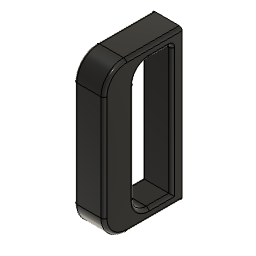
handle (Autodesk Fusion 360 design; units mm, degrees)
Autodesk Fusion 360 part; units mm, degrees
sketch "Sketch1" plane through (0, 0, 0) normal (1, 0, 0) x (0, 1, 0)
  line L0 (-66.04, 63.5) -> (0, 63.5)
  line L1 (0, 63.5) -> (0, -63.5)
  line L2 (0, -63.5) -> (-66.04, -63.5)
  line L3 (-66.04, -63.5) -> (-66.04, 63.5)
  line L4 (-8.89, 54.61) -> (-40.64, 54.61)
  line L5 (-40.64, 54.61) -> (-40.64, -54.61)
  line L6 (-40.64, -54.61) -> (-8.89, -54.61)
  line L7 (-8.89, -54.61) -> (-8.89, 54.61)
  dimension "d1" = 127
  dimension "d2" = 31.75
  dimension "d3" = 8.89
  dimension "d4" = 8.89
  dimension "d5" = 25.4
  dimension "d6" = 8.89
  constraint horizontal L0
  constraint vertical L1
  constraint horizontal L2
  constraint vertical L3
  constraint midpoint L1 origin
  constraint horizontal L4
  constraint vertical L5
  constraint horizontal L6
  constraint vertical L7
  measures "d1" distance of L0.end L1.end
  measures "d2" distance of L5 L7
  measures "d3" distance of L0 L4
  measures "d4" distance of L1 L7
  measures "d5" distance of L3 L5
  measures "d6" distance of L2 L6
extrude "Extrude1" add sketch "Sketch1" along normal mid plane 25.4
fillet "Fillet1" radius 12.7 1 edges at (0, -40.64, -54.61)
fillet "Fillet2" radius 12.7 1 edges at (0, -40.64, 54.61)
fillet "Fillet3" radius 19.05 1 edges at (0, -66.04, 63.5)
fillet "Fillet4" radius 19.05 1 edges at (0, -66.04, -63.5)
sketch "Sketch2" plane through (0, -66.04, 0) normal (0, -1, 0) x (1, 0, 0)
  line L0 (-12.7, -44.45) -> (12.7, -44.45)
  line L1 (12.7, -44.45) -> (12.7, 44.45)
  line L2 (12.7, 44.45) -> (-12.7, 44.45)
  line L3 (-12.7, 44.45) -> (-12.7, -44.45)
  line L4 (7.181, -50.5634) -> (7.181, 50.5634) construction
  line L5 (7.181, 50.5634) -> (-7.181, 50.5634) construction
  line L6 (-7.181, 50.5634) -> (-7.181, -50.5634) construction
  line L7 (-7.181, -50.5634) -> (7.181, -50.5634) construction
  dimension "d17" = 12.7
  constraint vertical L6
  constraint horizontal origin
  constraint vertical origin
extrude "Extrude2" [suppressed]
fillet "Fillet5" radius 2.5 23 edges at (12.7, -8.89, 0) (0, -8.89, 54.61) (12.7, -18.415, -54.61) (12.7, -36.9203, -50.8903) (12.7, -40.64, 0) (12.7, -36.9203, 50.8903) (12.7, -18.415, 54.61) (-12.7, -8.89, 0) (-12.7, -18.415, 54.61) (-12.7, -36.9203, 50.8903) (-12.7, -40.64, 0) (-12.7, -36.9203, -50.8903) (-12.7, -18.415, -54.61) (12.7, -23.495, 63.5) (12.7, -60.4604, 57.9204) (12.7, -66.04, 0) (12.7, -60.4604, -57.9204) (12.7, -23.495, -63.5) (-12.7, -23.495, 63.5) (-12.7, -60.4604, 57.9204) (-12.7, -66.04, 0) (-12.7, -60.4604, -57.9204) (-12.7, -23.495, -63.5)
